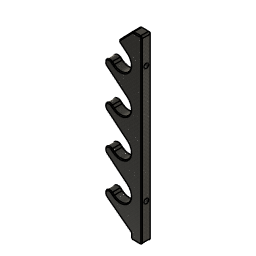
Porta vara v1 (Autodesk Fusion 360 design; units mm, degrees)
Autodesk Fusion 360 part; units mm, degrees
sketch "Sketch2" plane through (0, 0, 0) normal (0, 1, 0) x (1, 0, 0)
  line L0 (72.2479, 112.6909) -> (72.2479, -118.3289)
  line L1 (72.2479, 112.6909) -> (58.6479, 112.6909)
  line L2 (58.6479, 112.6909) -> (58.6479, 105.2312)
  line L3 (58.6479, 105.2312) -> (27.4854, 81.5611)
  arc A0 (27.4854, 81.5611) -> (33.8891, 73.4625) centre (30.6085, 77.4495) ccw
  line L4 (33.8891, 73.4625) -> (36.3566, 75.4929)
  arc A1 (53.5122, 54.6437) -> (36.3566, 75.4929) centre (44.9344, 65.0683) ccw
  line L5 (53.5122, 54.6437) -> (27.4854, 33.2278)
  line L6 (53.5122, 6.3104) -> (27.4854, -15.1055)
  arc A2 (53.5122, 6.3104) -> (36.3566, 27.1595) centre (44.9344, 16.735) ccw
  line L7 (53.5122, -42.0229) -> (27.4854, -63.4389)
  arc A3 (53.5122, -42.0229) -> (36.3566, -21.1738) centre (44.9344, -31.5984) ccw
  line L8 (53.5122, -90.3563) -> (27.4854, -111.7722)
  arc A4 (53.5122, -90.3563) -> (36.3566, -69.5071) centre (44.9344, -79.9317) ccw
  line L9 (72.2479, -118.3289) -> (60.5082, -118.3289)
  line L10 (60.5082, -118.3289) -> (43.0561, -100.3082)
  line L11 (43.0561, -100.3082) -> (43.0561, -98.96)
  line L12 (33.8891, 25.1292) -> (36.3566, 27.1595)
  arc A5 (27.4854, 33.2278) -> (33.8891, 25.1292) centre (30.6085, 29.1162) ccw
  line L13 (33.8891, -23.2041) -> (36.3566, -21.1738)
  arc A6 (27.4854, -15.1055) -> (33.8891, -23.2041) centre (30.6085, -19.2171) ccw
  line L14 (33.8891, -71.5375) -> (36.3566, -69.5071)
  arc A7 (27.4854, -63.4389) -> (33.8891, -71.5375) centre (30.6085, -67.5505) ccw
  dimension "d3" = 128
  dimension "d5" = 27
  dimension "d8" = 0
  dimension "d9" = -145
  constraint vertical L0
  constraint perpendicular L0 L1
  constraint perpendicular L1 L2
  constraint tangent L3 A0
  constraint tangent A0 L4
  constraint tangent L4 A1
  constraint parallel L4 L5
  constraint tangent A1 L5
  constraint perpendicular L0 L9
  constraint coincident L8 L11.end
  constraint perpendicular L9 L11
  measures "d5" distance of A0.end L5
extrude "Extrude1" add sketch "Sketch2" along normal blind 12
sketch "Sketch3" plane through (72.2479, 0, 0) normal (1, 0, 0) x (0, 1, 0)
  line L0 (0, 118.3289) -> (0, -112.6909)
  line L1 (0, -112.6909) -> (12, -112.6909)
  line L2 (12, -112.6909) -> (12, 118.3289)
  line L3 (12, 118.3289) -> (0, 118.3289)
  line L4 (0, 83.4322) -> (12, 83.4322) construction
  circle A0 centre (6, 83.4322) radius 3
  line L5 (0, -66.5678) -> (12, -66.5678) construction
  circle A1 centre (6, -66.5678) radius 3
  dimension "d12" = 6
  dimension "d13" = 150
  constraint coincident L0 L4.start
  constraint coincident L2 L4.end
  constraint perpendicular L2 L4
  constraint midpoint L4 A0.centre
  constraint coincident L0 L5.start
  constraint coincident L2 L5.end
  constraint perpendicular L2 L5
  constraint midpoint L5 A1.centre
  constraint equal A0 A1
  measures "d12" diameter of A0
  measures "d13" distance of L4 L5
extrude "Extrude2" cut sketch "Sketch3" against normal blind 40 contours A0 | A1
chamfer "Chamfer1" distance 2.5 distance2 1 2 edges at (58.4251, 6, 80.4322) (57.6625, 6, -69.5678) measured on face at (55.6331, 5.9785, 88.1649) measured on face at (58.0899, 5.9853, -62.0383)
fillet "Fillet1" radius 2 7 edges at (58.6479, 6, -105.2312) (58.6479, 6, -112.6909) (72.2479, 6, -112.6909) (72.2479, 6, 118.3289) (60.5082, 6, 118.3289) (43.0561, 6, 100.3082) (43.0561, 6, 98.96)
chamfer "Chamfer2" distance 1 distance2 1 56 edges at (51.8784, 0, 109.418) (43.278, 0, 99.6115) (48.7581, 0, 94.2681) (55.3589, 0, 71.3539) (35.1229, 0, 70.5223) (26.5584, 0, 70.7529) (40.4988, 0, -43.9358) (55.3589, 0, -73.6461) (35.1229, 0, -74.4777) (26.5584, 0, -74.2471) (42.6716, 0, -93.096) (58.4395, 0, -105.3346) (58.6479, 0, -108.4572) (59.2337, 0, -112.1051) (65.4479, 0, -112.6909) (71.6621, 0, -112.1051) (72.2479, 0, 2.819) (71.6621, 0, 117.7431) (65.8017, 0, 118.3289) (60.5753, 0, 118.1704) (26.5584, 0, -25.9137) (35.1229, 0, -26.1444) (55.3589, 0, -25.3128) (40.4988, 0, 4.3976) (40.4988, 12, 4.3976) (26.5584, 12, -25.9137) (35.1229, 12, -26.1444) (55.3589, 12, -25.3128) (40.4988, 12, -43.9358) (26.5584, 12, 70.7529) (35.1229, 12, 70.5223) (55.3589, 12, 71.3539) (48.7581, 12, 94.2681) (43.278, 12, 99.6115) (51.8784, 12, 109.418) (60.5753, 12, 118.1704) (65.8017, 12, 118.3289) (71.6621, 12, 117.7431) (72.2479, 12, 2.819) (71.6621, 12, -112.1051) (65.4479, 12, -112.6909) (59.2337, 12, -112.1051) (58.6479, 12, -108.4572) (58.4395, 12, -105.3346) (42.6716, 12, -93.096) (26.5584, 12, -74.2471) (35.1229, 12, -74.4777) (55.3589, 12, -73.6461) (40.4988, 12, 52.7309) (26.5584, 12, 22.4196) (35.1229, 12, 22.189) (55.3589, 12, 23.0206) (40.4988, 0, 52.7309) (26.5584, 0, 22.4196) (35.1229, 0, 22.189) (55.3589, 0, 23.0206) measured on face at (67.6428, 0, -3.7679) measured on face at (43.2849, 8, 99.5218) measured on face at (50.3427, 4, 92.9643) measured on face at (67.6428, 0, -3.7679) measured on face at (34.7116, 4, 70.8607) measured on face at (25.5354, 8, 68.5112) measured on face at (44.8366, 4, -47.5051) measured on face at (67.6428, 0, -3.7679) measured on face at (34.7116, 4, -74.1393) measured on face at (25.4721, 8, -77.9751) measured on face at (47.7336, 4, -96.941) measured on face at (58.6, 4, -105.7885) measured on face at (58.6479, 4, -109.2018) measured on face at (58.9159, 4, -111.6909) measured on face at (67.0479, 4, -112.6909) measured on face at (72.2117, 4, -111.0694) measured on face at (67.6428, 0, -3.7679) measured on face at (70.6264, 4, 118.2927) measured on face at (67.6428, 0, -3.7679) measured on face at (60.6581, 4, 118.2033) measured on face at (25.4499, 8, -28.8963) measured on face at (34.7116, 4, -25.806) measured on face at (67.6428, 0, -3.7679) measured on face at (44.8366, 4, 0.8282) measured on face at (67.6428, 12, -3.7679) measured on face at (67.6428, 12, -3.7679) measured on face at (67.6428, 12, -3.7679) measured on face at (67.6428, 12, -3.7679) measured on face at (67.6428, 12, -3.7679) measured on face at (67.6428, 12, -3.7679) measured on face at (67.6428, 12, -3.7679) measured on face at (67.6428, 12, -3.7679) measured on face at (67.6428, 12, -3.7679) measured on face at (43.2849, 8, 99.5218) measured on face at (67.6428, 12, -3.7679) measured on face at (60.6581, 4, 118.2033) measured on face at (67.6428, 12, -3.7679) measured on face at (70.6264, 4, 118.2927) measured on face at (67.6428, 12, -3.7679) measured on face at (72.2117, 4, -111.0694) measured on face at (67.6428, 12, -3.7679) measured on face at (58.9159, 4, -111.6909) measured on face at (67.6428, 12, -3.7679) measured on face at (58.6, 4, -105.7885) measured on face at (67.6428, 12, -3.7679) measured on face at (67.6428, 12, -3.7679) measured on face at (67.6428, 12, -3.7679) measured on face at (67.6428, 12, -3.7679) measured on face at (67.6428, 12, -3.7679) measured on face at (67.6428, 12, -3.7679) measured on face at (67.6428, 12, -3.7679) measured on face at (67.6428, 12, -3.7679) measured on face at (44.8366, 4, 49.1616) measured on face at (26.1685, 8, 16.5817) measured on face at (34.7116, 4, 22.5273) measured on face at (67.6428, 0, -3.7679)
